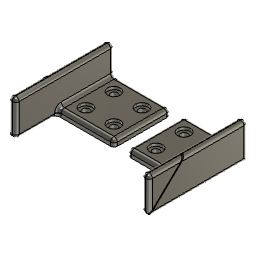
_paper guides.c25c2183-df1f-4a5f-b5f6-c267c81911b1 (Autodesk Fusion 360 design; units mm, degrees)
Autodesk Fusion 360 part; units mm, degrees
note: some values were not read from the file. Chosen so that the rebuilt part matches the saved one: which face or edge a step refers to; which pieces of a blend or face edit are solid. Set by a fixed rule: which sketch regions a step uses.
sketch "Sketch1" plane through (0, 0, 0) normal (0, 0, 1) x (1, 0, 0)
  line L0 (0, 0) -> (45, 0)
  line L1 (45, 0) -> (45, 40)
  line L2 (45, 40) -> (0, 40)
  line L3 (0, 40) -> (0, 0)
  dimension "d1" = 45
  dimension "d2" = 40
  constraint horizontal L0
  constraint vertical L1
  constraint horizontal L2
  constraint vertical L3
  constraint coincident L0.start L3.end
  measures "d1" distance of L0.start L0.end
  measures "d2" distance of L0.start L2.end
extrude "Extrude1" add sketch "Sketch1" along normal blind 5 makes body 1
sketch "Sketch2" plane through (0, 0, 5) normal (0, 0, 1) x (-1, 0, 0)
  line L0 (0, -40) -> (0, 0)
  line L1 (0, 0) -> (-45, 0)
  line L2 (-45, 0) -> (-45, -40)
  line L3 (-45, -40) -> (0, -40)
  circle A0 centre (-10, -30) radius 2.5
  circle A1 centre (-10, -10) radius 2.5
  circle A2 centre (-30, -10) radius 2.5
  circle A3 centre (-30, -30) radius 2.5
  dimension "d5" = 5
  dimension "d6" = 5
  dimension "d7" = 5
  dimension "d8" = 5
  measures "d5" diameter of A0
  measures "d6" diameter of A1
  measures "d7" diameter of A2
  measures "d8" diameter of A3
extrude "Extrude2" cut sketch "Sketch2" against normal blind 5 contours A0 | A1 | A2 | A3 bodies 1
sketch "Sketch3" plane through (0, 0, 5) normal (0, 0, 1) x (-1, 0, 0)
  circle A0 centre (-10, -10) radius 2.5
  circle A1 centre (-30, -10) radius 2.5
  circle A2 centre (-10, -30) radius 2.5
  circle A3 centre (-30, -30) radius 2.5
  line L0 (0, -40) -> (0, 0)
  line L1 (0, 0) -> (-45, 0)
  line L2 (-45, 0) -> (-45, -40)
  line L3 (-45, -40) -> (0, -40)
  line L4 (-45, -40) -> (-40, -40)
  line L5 (-40, -40) -> (-40, 0)
  line L6 (-40, 0) -> (-45, 0)
  line L7 (-45, 0) -> (-45, -40)
  dimension "d11" = 5
  dimension "d12" = 40
  constraint horizontal L4
  constraint vertical L5
  constraint horizontal L6
  constraint vertical L7
  constraint coincident L2.end L3.start
  measures "d11" distance of L2.end L4.end
  measures "d12" distance of L2.end L1.end
extrude "Extrude3" add sketch "Sketch3" along normal blind 20 contours L1 L2 L3 L4 L5 L6 L7 bodies 1
sketch "Sketch4" plane through (0, 0, 0) normal (0, -1, 0) x (1, 0, 0)
  line L0 (0, 0) -> (45, 0)
  line L1 (45, 0) -> (45, 25)
  line L2 (45, 25) -> (40, 25)
  line L3 (40, 25) -> (40, 5)
  line L4 (40, 5) -> (0, 5)
  line L5 (0, 5) -> (0, 0)
  line L6 (40, 25) -> (45, 25)
  line L7 (45, 25) -> (45, 0)
  line L8 (45, 0) -> (40, 0)
  line L9 (40, 0) -> (40, 25)
  constraint horizontal L6
  constraint vertical L7
  constraint horizontal L8
  constraint vertical L9
  constraint coincident L0.end L1.start
  constraint coincident L2.end L3.start
extrude "Extrude4" add sketch "Sketch4" along normal blind 30 contours L0 L1 L2 L3 L6 L7 L8 L9 bodies 1
sketch "Sketch5" plane through (45, 0, 0) normal (1, 0, 0) x (0, 1, 0)
  line L0 (-30, 0) -> (40, 0)
  line L1 (40, 0) -> (40, 25)
  line L2 (40, 25) -> (-30, 25)
  line L3 (-30, 25) -> (-30, 0)
  line L4 (-31, 0) -> (-4, 26)
  line L5 (-4, 26) -> (-3.5189, 25.5004)
  line L6 (-3.5189, 25.5004) -> (-30.5189, -0.4996)
  line L7 (-30.5189, -0.4996) -> (-31, 0)
  constraint perpendicular L4 L5
  constraint parallel L4 L6
  constraint parallel L5 L7
extrude "Extrude5" cut sketch "Sketch5" against normal blind 2 contours L2 L3 L4 L6 | L2 L4 L5 L6 bodies 1
fillet "Fillet1" radius 2.4 20 edges at (41.5, -30, 0) (44, -30, 0) (40, -30, 12.5) (45, -30, 12.9815) (42.5, -30, 25) (40, 5, 25) (45, -17.5192, 25) (45, 17.9808, 25) (45, 5, 0) (45, 40, 12.5) (42.5, 40, 25) (40, 40, 15) (20, 40, 5) (20, 0, 5) (0, 20, 5) (40, 20, 5) (40, -15, 0) (0, 40, 2.5) (0, 0, 2.5) (40, 0, 2.5) on bodies 1
sketch "Sketch6" plane through (0, 0, 5) normal (0, 0, 1) x (-1, 0, 0)
  circle A0 centre (-30, -30) radius 2.5
  circle A1 centre (-10, -30) radius 2.5
  circle A2 centre (-30, -10) radius 2.5
  circle A3 centre (-10, -10) radius 2.5
  line L0 (-37.6, -2.4) -> (-37.6, -37.6)
  line L1 (-37.6, -37.6) -> (-2.4, -37.6)
  line L2 (-2.4, -37.6) -> (-2.4, -2.4)
  line L3 (-2.4, -2.4) -> (-37.6, -2.4)
  circle A4 centre (-10, -30) radius 4.5
  circle A5 centre (-30, -30) radius 4.5
  circle A6 centre (-10, -10) radius 4.5
  circle A7 centre (-30, -10) radius 4.5
  dimension "d21" = 9
  dimension "d22" = 9
  dimension "d23" = 9
  dimension "d24" = 9
  constraint concentric A1 A4
  constraint concentric A0 A5
  constraint concentric A3 A6
  constraint concentric A2 A7
  measures "d21" diameter of A4
  measures "d22" diameter of A5
  measures "d23" diameter of A6
  measures "d24" diameter of A7
extrude "Extrude6" cut sketch "Sketch6" against normal blind 2 contours A4 | A5 | A6 | A7 bodies 1
move_body "Move1" bodies 1 to x (1, 0, 0) y (0, 1, 0) z (0, 0, 1) at (5, 0, 0)
mirror "Mirror1" about plane through (0, 0, 0) normal (1, 0, 0) of bodies 1 makes body 2
